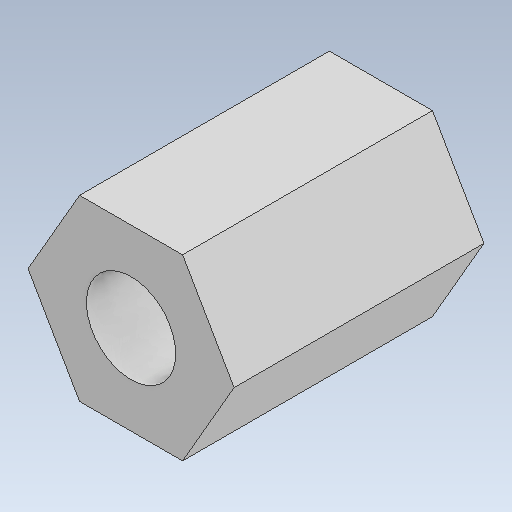
# Autodesk Inventor part: M2.5x7mm_Standoff_ 970070151
Saved by Autodesk Inventor 2021 (Build 250183000, 183)
## iProperties
Created: 2020-06-14
Part Number: M2.5x7mm_Standoff_ 970070151
Material: Generic
Document SubType Name: Modeling
Designer: Viktor Lindström
Density: 1 g/cm^3
Appearance: Default
Author: Viktor Lindström
Autodesk Inventor part; units mm, degrees
ref_plane "YZ Plane" through (0, 0, 0) normal (1, 0, 0) x (0, 1, 0)
ref_plane "XZ Plane" through (0, 0, 0) normal (0, 1, 0) x (-1, 0, 0)
ref_plane "XY Plane" through (0, 0, 0) normal (0, 0, 1) x (1, 0, 0)
sketch "Sketch1" plane through (0, 0, 0) normal (0, 0, 1) x (1, 0, 0)
  line L0 (2.8868, 0) -> (1.4434, -2.5)
  line L1 (1.4434, -2.5) -> (-1.4434, -2.5)
  line L2 (-1.4434, -2.5) -> (-2.8868, 0)
  line L3 (-2.8868, 0) -> (-1.4434, 2.5)
  line L4 (-1.4434, 2.5) -> (1.4434, 2.5)
  line L5 (1.4434, 2.5) -> (2.8868, 0)
  point P0 (0, 0)
  point P1 (0, 0)
  dimension "d0" = 5
  constraints: 12 end point, 1 coincident, 13 other
  measures "d0" distance between parallel lines of L4 L1
extrude "Extrusion1" add sketch "Sketch1" along normal blind 7
sketch "Sketch3" plane through (0, 0, 0) normal (0, 0, -1) x (-1, 0, 0)
  circle A0 centre (0, 0) radius 1.25
  dimension "d6" = 2.5
  constraints: 1 centre point, 1 coincident
  measures "d6" diameter of A0
extrude "Extrusion3" cut sketch "Sketch3" against normal through all
body "Solid1"
